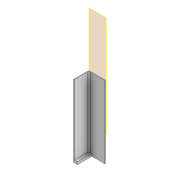
# Autodesk Inventor part: 50_Nema12_Linearmotor_150mm_cage
Saved by Autodesk Inventor 2022 (Build 260153000, 153)
## iProperties
Created: 2023-03-17
Part Number: 50_Nema12_Linearmotor_150mm_cage
Material: Generisch
Document SubType Name: Modeling
Designer: diederichbenedict
Density: 1 g/cm^3
Appearance: Vorgabe
Author: diederichbenedict
Autodesk Inventor part; units mm, degrees
ref_plane "YZ Plane" through (0, 0, 0) normal (1, 0, 0) x (0, 1, 0)
ref_plane "XZ Plane" through (0, 0, 0) normal (0, 1, 0) x (-1, 0, 0)
ref_plane "XY Plane" through (0, 0, 0) normal (0, 0, 1) x (1, 0, 0)
ref_plane "Arbeitsebene1" through (0, 0, 0) normal (0, 0, 1) x (1, 0, 0)
sketch "Skizze1" plane through (0, 0, 0) normal (0, 0, 1) x (1, 0, 0)
  line L0 (0, 0) -> (-35, 0)
  line L1 (-35, 0) -> (-35, -150)
  line L2 (-35, -150) -> (0, -150)
  line L3 (0, -150) -> (0, 0)
  dimension "d18" = 35
  dimension "d19" = 150
  constraints: 8 end point, 2 parallel, 1 horizontal, 1 perpendicular
  measures "d18" distance of L2.end L1.end
  measures "d19" distance of L1.end L0.end
extrude "Extrusion1" add sketch "Skizze1" along normal blind 1.5
sketch "Skizze2" plane through (0, 0, 1.5) normal (0, 0, 1) x (1, 0, 0)
  line L0 (-35, 0) -> (-35, -150) projected
  line L1 (0, 0) -> (-35, 0) projected
  line L2 (0, -150) -> (0, 0) projected
  line L3 (-35, -150) -> (0, -150) projected
  line L4 (0, 0) -> (-35, 0) projected
  line L5 (-35, -150) -> (-33.5, -150)
  line L6 (-33.5, -150) -> (-33.5, 0)
  line L7 (-33.5, 0) -> (-35, 0)
  line L8 (-35, 0) -> (-35, -150)
  point P0 (0, -87)
  point P1 (-33.5, 0)
  dimension "d20" = 1.5
  constraints: 8 end point, 2 parallel, 1 horizontal, 1 perpendicular, 1 point on line
  measures "d20" distance of L7.end L6.end
extrude "Extrusion2" add sketch "Skizze2" along normal blind 30 contours L1 L6 L3 L0
fillet "Rundung2" radius 3 2 edges at (-35, -75, 0) (-33.5, -75, 1.5)
sketch "Skizze6" plane through (-33.5, -150, 31.5) normal (1, 0, 0) x (0, 0, -1)
  line L0 (31.5, 0) -> (31.5, 150) projected
  line L1 (0, 0) -> (31.5, 0)
  line L2 (31.5, 0) -> (31.5, 5)
  line L3 (31.5, 5) -> (0, 5)
  line L4 (0, 5) -> (0, 0)
  line L5 (30.1312, 5) -> (30.1312, 0)
  dimension "d22" = 5
  constraints: 10 end point, 3 parallel, 3 point on line, 1 horizontal, 1 perpendicular
  measures "d22" distance of L2.end L1.end
extrude "Extrusion6" add sketch "Skizze6" along normal blind 6.5 contours L1 L4 L3 L5
